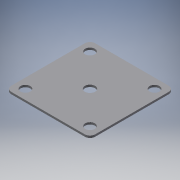
# Autodesk Inventor part: Part_Metal
Saved by Autodesk Inventor 2019 (Build 230136000, 136)
## iProperties
Created: 2019-04-26
Part Number: Part_Metal
Material: 일반
Document SubType Name: Modeling
Designer: hinmo
Density: 1 g/cm^3
Appearance: 기본값
Author: hinmo
Autodesk Inventor part; units mm, degrees
ref_plane "YZ Plane" through (0, 0, 0) normal (1, 0, 0) x (0, 1, 0)
ref_plane "XZ Plane" through (0, 0, 0) normal (0, 1, 0) x (-1, 0, 0)
ref_plane "XY Plane" through (0, 0, 0) normal (0, 0, 1) x (1, 0, 0)
sketch "스케치1" plane through (0, 0, 0) normal (0, 1, 0) x (-1, 0, 0)
  line L0 (-36, 41) -> (36, 41)
  line L1 (41, 36) -> (41, -36)
  line L2 (36, -41) -> (-36, -41)
  line L3 (-41, -36) -> (-41, 36)
  line L4 (-41, 41) -> (41, -41) construction
  line L5 (41, 41) -> (-41, -41) construction
  arc A0 (41, 36) -> (36, 41) centre (36, 36) ccw
  arc A1 (-36, 41) -> (-41, 36) centre (-36, 36) ccw
  arc A2 (-41, -36) -> (-36, -41) centre (-36, -36) ccw
  arc A3 (36, -41) -> (41, -36) centre (36, -36) ccw
  line L6 (-26.75, 31.5) -> (26.75, 31.5)
  line L7 (31.5, 26.75) -> (31.5, -26.75)
  line L8 (26.75, -31.5) -> (-26.75, -31.5)
  line L9 (-31.5, -26.75) -> (-31.5, 26.75)
  line L10 (-31.5, 31.5) -> (31.5, -31.5) construction
  line L11 (31.5, 31.5) -> (-31.5, -31.5) construction
  circle A4 centre (31.5, -31.5) radius 4.75
  circle A5 centre (31.5, 31.5) radius 4.75
  circle A6 centre (-31.5, 31.5) radius 4.75
  circle A7 centre (-31.5, -31.5) radius 4.75
  circle A8 centre (0, 0) radius 5
  dimension "d0" = 82
  dimension "d1" = 82
  dimension "d2" = 5
  dimension "d3" = 63
  dimension "d4" = 63
  dimension "d5" = 9.5
  dimension "d6" = 9.5
  dimension "d7" = 9.5
  dimension "d8" = 9.5
  dimension "d9" = 10
  constraints: 24 end point, 16 point on circle, 9 centre point, 8 point on line, 8 tangent, 4 midpoint, 4 parallel, 3 equal radius, 2 coincident, 2 horizontal, 2 perpendicular
  measures "d0" distance of L4.end L5.end
  measures "d1" distance of L5.start L4.end
  measures "d2" radius of A0
  measures "d3" distance of L10.end L11.end
  measures "d4" distance of L11.start L10.end
  measures "d5" diameter of A4
  measures "d6" diameter of A5
  measures "d7" diameter of A6
  measures "d8" diameter of A7
  measures "d9" diameter of A8
extrude "돌출1" add sketch "스케치1" along normal blind 2 contours L0 A0 L1 A3 L2 A2 L3 A1 | L6 A5 L7 A4 L8 A7 L9 A6
